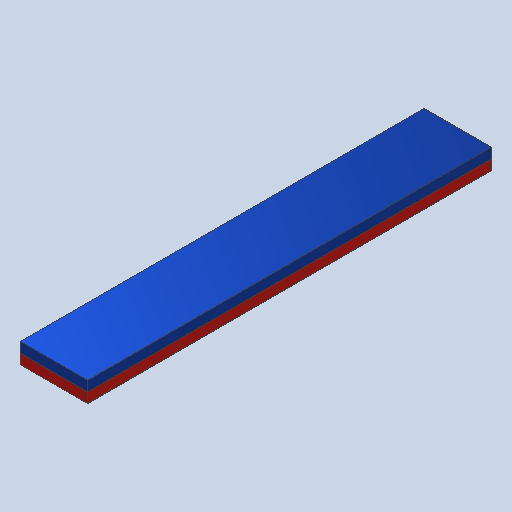
# Autodesk Inventor part: HalbachMagnet
Saved by Autodesk Inventor 2022.2 (Build 262287000, 287)
## iProperties
Created: 2022-07-28
Part Number: HalbachMagnet
Material: Generic
Document SubType Name: Modeling
Designer: ABL
Density: 1 g/cm^3
Appearance: Default
Author: ABL
Autodesk Inventor part; units mm, degrees
ref_plane "YZ Plane" through (0, 0, 0) normal (1, 0, 0) x (0, 1, 0)
ref_plane "XZ Plane" through (0, 0, 0) normal (0, 1, 0) x (-1, 0, 0)
ref_plane "XY Plane" through (0, 0, 0) normal (0, 0, 1) x (1, 0, 0)
sketch "Sketch1" plane through (0, 0, 0) normal (0, 1, 0) x (-1, 0, 0)
  line L0 (0, 0) -> (-10, 0)
  line L1 (-10, 0) -> (-10, -60)
  line L2 (-10, -60) -> (0, -60)
  line L3 (0, -60) -> (0, 0)
  dimension "d0" = 10
  dimension "d1" = 60
  constraints: 8 end point, 2 parallel, 1 horizontal, 1 perpendicular
  measures "d0" distance of L2.end L1.end
  measures "d1" distance of L1.end L0.end
extrude "Extrusion1" add sketch "Sketch1" along normal blind 1.5
chamfer "Chamfer1" distance 0.002 angle 45 8 edges at (5, 0, -60) (0, 0, -30) (5, 0, 0) (10, 0, -30) (10, 0.75, -60) (0, 0.75, -60) (0, 0.75, 0) (10, 0.75, 0)
extrude "Extrusion2" add sketch "Sketch1" against normal blind 1.5
equation "\"d0\" = halbachMagnet_width"
equation "\"d1\" = halbachMagnet_length"
equation "\"d2\" = 0.5 * halbachMagnet_height"
equation "\"d7\" = 0.5 * halbachMagnet_height"
equation "\"gap\" = 0.1"
equation "\"airgap\" = 0.4"
equation "\"driveMagnet_height\" = 5"
equation "\"halbachMagnet_length\" = 60"
equation "\"halbachMagnet_width\" = 10"
equation "\"halbachMagnet_height\" = 3"
equation "\"sensorMagnet_diameter\" = 5"
equation "\"sensorMagnet_height\" = 2.66667"
equation "\"wallgap\" = 2"
equation "\"motorRadius\" = 2 * gap + driveMagnet_centerSpacingRadius + driveMagnet_length + 2 * wallgap"
equation "\"shaftDiameter\" = 8"
equation "\"flangeBearing_outerDiameter\" = 16"
equation "\"flangeBearing_innerDiameter\" = shaftDiameter"
equation "\"flangeBearing_height\" = 5"
equation "\"flangeBearing_flangeHeight\" = 1"
equation "\"flangeBearing_flangeDiameter\" = 18"
equation "\"magnetTrapNut_height\" = 1.2"
equation "\"magnetTrapNut_sideToSide\" = 4"
equation "\"magnetTrapBolt_headHeight\" = 2"
equation "\"magnetTrapBolt_headDiameter\" = 3.98"
equation "\"magnetTrapBolt_diameter\" = 2"
equation "\"statorThickness\" = coilThickness + 2 * wallgap"
equation "\"rotor_mountingLipHeight\" = 0.5 * statorThickness"
equation "\"magnetTrapHexNut_sideToSide\" = 4"
equation "\"magnetTrapSquareNut_sideLength\" = 4"
equation "\"magnetTrapSquareNut_height\" = 1.2"
equation "\"magnetTrapHexNut_height\" = 1.2"
equation "\"rotorRadius\" = 2 * gap + driveMagnet_centerSpacingRadius + driveMagnet_length + wallgap"
equation "\"rotorBandSquareNut_sideLength\" = 4"
equation "\"rotorBandHexNut_height\" = 1.2"
equation "\"rotorBandHexNut_sideToSide\" = 4"
equation "\"rotorBandSquareNut_height\" = 1.2"
equation "\"rotorBandBolt_headHeight\" = 2"
equation "\"rotorBandBolt_headDiameter\" = 3.98"
equation "\"rotorBandBolt_diameter\" = 2"
equation "\"rotorBandThickness\" = wallgap + rotorBandBolt_headHeight + gap"
equation "\"flangeCoupling_collarOuterDiameter\" = 16"
equation "\"flangeCoupling_flangeHoleEdgeToEdge\" = 2.05"
equation "\"flangeCoupling_innerDiameter\" = shaftDiameter"
equation "\"flangeCoupling_flangeHoleDiameter\" = 3.9"
equation "\"flangeCoupling_flangeHeight\" = 3.1"
equation "\"flangeCoupling_flangeDiameter\" = 32"
equation "\"flangeCoupling_height\" = flangeCoupling_collarHeight + flangeCoupling_flangeHeight"
equation "\"flangeCoupling_mountHoleDiameter\" = 3.9"
equation "\"flangeCoupling_mountHoleEdgeToEdge\" = 2.05"
equation "\"statorRadius\" = driveMagnet_length + driveMagnet_centerSpacingRadius + 2 * gap"
equation "\"statorMountBolt_diameter\" = 4"
equation "\"statorMountBolt_headDiameter\" = 7"
equation "\"statorMountBolt_headHeight\" = 4"
equation "\"statorMountBolt_shaftLength\" = coilThickness + flangeCoupling_flangeHeight + wallgap"
equation "\"statorMountHexNut_height\" = 4"
equation "\"statorMountHexNut_sideToSide\" = 8"
equation "\"sensorMagnet_ringRadius\" = 0.5 * driveMagnet_centerSpacingRadius + 2 * wallgap"
equation "\"coil_percentCoverage\" = 0.6"
equation "\"statorSpokeDegrees\" = 4deg"
equation "\"coil_bulge\" = 3"
equation "\"statorCoilHexNut_height\" = 1.2"
equation "\"statorCoilBolt_headHeight\" = 2"
equation "\"statorCoilBolt_diameter\" = 2"
equation "\"statorCoilBolt_headDiameter\" = 3.98"
equation "\"statorCoilHexNut_sideToSide\" = 4"
equation "\"driveMagnet_centerSpacingRadius\" = 38.96113"
equation "\"driveMagnet_length\" = 60"
equation "\"coilThickness\" = 10"
equation "\"flangeCoupling_collarHeight\" = 10"
body "Solid1"
